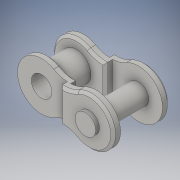
# Autodesk Inventor part: HalfLink
Saved by Autodesk Inventor 2016 (Build 200138000, 138)
## iProperties
Created: 2016-10-03
Part Number: HalfLink
Material: Generic
Document SubType Name: Modeling
Designer: Kevin G
Density: 1 g/cm^3
Appearance: Default
Author: Kevin G
Autodesk Inventor part; units mm, degrees
ref_plane "YZ Plane" through (0, 0, 0) normal (1, 0, 0) x (0, 1, 0)
ref_plane "Work Plane1" through (0, 0, 3.6512) normal (0, 0, 1) x (1, 0, 0)
sketch "Sketch1" plane through (0, 0, 3.6512) normal (0, 0, 1) x (1, 0, 0)
  arc A0 (2.0955, 3.6295) -> (2.0955, -3.6295) centre (0, 0) ccw
  arc A1 (2.0955, 3.6295) -> (5.0478, 2.9225) centre (4.7625, 8.2489) ccw
  line L0 (5.0478, 2.9225) -> (5.0478, -2.9225)
  arc A2 (5.0478, -2.9225) -> (2.0955, -3.6295) centre (4.7625, -8.2489) ccw
  constraints: 6 point on circle, 3 centre point, 2 end point
extrude "Extrusion1" add sketch "Sketch1" against normal blind 1.27
chamfer "Chamfer1" distance 0.4233 angle 45 4 edges at (-4.191, 0, 2.3812) (3.5203, 3.0615, 2.3812) (5.0478, 0, 2.3812) (3.5203, -3.0615, 2.3812)
sketch "Sketch2" plane through (0, 0, 0) normal (0, 0, 1) x (1, 0, 0)
  circle A0 centre (0, 0) radius 2.54
  constraints: 1 centre point
extrude "Extrusion2" add sketch "Sketch2" along normal mid plane 6.0325
mirror "Mirror1" about plane through (0, 0, 0) normal (0, 0, 1) of "Extrusion1", "Chamfer1"
sketch "Sketch3" plane through (0, 0, 0) normal (0, 0, 1) x (1, 0, 0)
  circle A0 centre (0, 0) radius 1.7907
  constraints: 1 centre point
extrude "Extrusion3" cut sketch "Sketch3" along normal through all both and the other way through all
ref_plane "Work Plane2" through (0, 0, 4.9213) normal (0, 0, 1) x (1, 0, 0)
sketch "Sketch4" plane through (0, 0, 4.9213) normal (0, 0, 1) x (1, 0, 0)
  arc A0 (4.4772, 2.9225) -> (7.4295, 3.6295) centre (4.7625, 8.2489) ccw
  arc A1 (7.4295, -3.6295) -> (7.4295, 3.6295) centre (9.525, 0) ccw
  arc A2 (7.4295, -3.6295) -> (4.4772, -2.9225) centre (4.7625, -8.2489) ccw
  line L0 (4.4772, 2.9225) -> (4.4772, -2.9225)
  constraints: 6 point on circle, 3 centre point, 2 end point
extrude "Extrusion4" add sketch "Sketch4" against normal blind 1.27
chamfer "Chamfer2" distance 0.4233 angle 45 4 edges at (6.0047, 3.0615, 4.9213) (4.4772, 0, 4.9213) (6.0047, -3.0615, 4.9213) (13.716, 0, 4.9213)
mirror "Mirror2" about plane through (0, 0, 0) normal (0, 0, 1) of "Extrusion4", "Chamfer2"
sketch "Sketch5" plane through (0, 0, 0) normal (0, 0, 1) x (1, 0, 0)
  circle A0 centre (9.525, 0) radius 1.7907
  constraints: 1 centre point
extrude "Extrusion5" add sketch "Sketch5" along normal mid plane 11.1125
body "Solid1"
